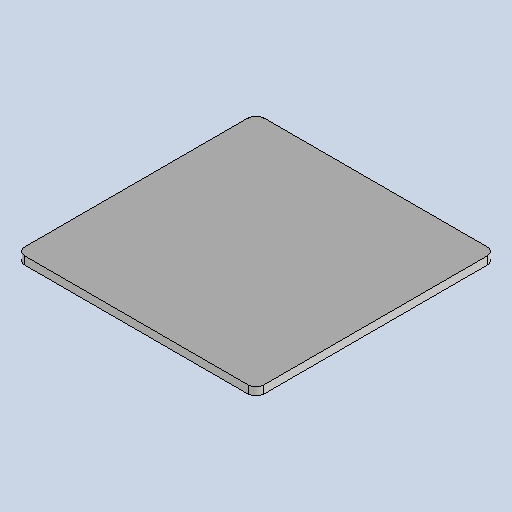
# Autodesk Inventor part: TZS 767 FDS 1200 CUP 2
Saved by Autodesk Inventor 2025.1 (Build 291241020, 241B)
## iProperties
Created: 2025-06-24
Part Number: TZS 767 FDS 1200 CUP 2
Material: Stainless Steel
Document SubType Name: Sheet Metal
Designer: user
Mass: 57.5451 g
Surface Area: 76.6627 cm^2
Volume: 7.19313 cm^3
Density: 8 g/cm^3
Flat Pattern Width: 6 cm
Flat Pattern Length: 6 cm
Flat Pattern Area: 36 cm^2
Sheet Metal Rule: AISI304 2mm Die16
Sheet Metal Width: 60.000 mm
Sheet Metal Length: 60.000 mm
Sheet Metal Area: 3600.000 mm^2
Appearance: Default
Author: user
Autodesk Inventor part; units mm, degrees
ref_plane "YZ Plane" through (0, 0, 0) normal (1, 0, 0) x (0, 1, 0)
ref_plane "XZ Plane" through (0, 0, 0) normal (0, 1, 0) x (-1, 0, 0)
ref_plane "XY Plane" through (0, 0, 0) normal (0, 0, 1) x (1, 0, 0)
sketch "Sketch1" plane through (0, 0, 0) normal (0, 0, 1) x (1, 0, 0)
  line L0 (-30, -30) -> (30, -30)
  line L1 (30, -30) -> (30, 30)
  line L2 (30, 30) -> (-30, 30)
  line L3 (-30, 30) -> (-30, -30)
  line L4 (-30, -30) -> (30, 30) construction
  line L5 (30, -30) -> (-30, 30) construction
  line L6 (15.25, -15.25) -> (-15.25, -15.25)
  line L7 (-15.25, -15.25) -> (-15.25, 15.25)
  line L8 (-15.25, 15.25) -> (15.25, 15.25)
  line L9 (15.25, 15.25) -> (15.25, -15.25)
  line L10 (15.25, -15.25) -> (-15.25, 15.25) construction
  line L11 (-15.25, -15.25) -> (15.25, 15.25) construction
  point P0 (0, 0)
  dimension "d154" = 60
  dimension "d155" = 60
  dimension "d172" = 30.5
  measures "d154" distance of L1.end L2.end
  measures "d155" distance of L0.end L1.end
  measures "d172" distance of L7.end L8.end
extrude "Plate5" add sketch "Sketch1" along normal blind 2 contours L3 L2 L1 L0 | L6 L7 L8 L9
fillet "Corner Round1" radius 2 4 edges at (30, 30, 1) (-30, 30, 1) (-30, -30, 1) (30, -30, 1)
body "Solid3"
